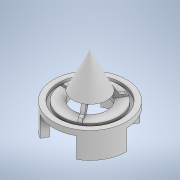
# Autodesk Inventor part: Reflector+feet
Saved by Autodesk Inventor 2022.4 (Build 264492010, 492A)
## iProperties
Created: 2022-12-05
Part Number: Reflector+feet
Material: Generic
Document SubType Name: Modeling
Designer: tmass
Density: 1 g/cm^3
Appearance: Default
Author: tmass
Autodesk Inventor part; units mm, degrees
ref_plane "YZ Plane" through (0, 0, 0) normal (1, 0, 0) x (0, 1, 0)
ref_plane "XY Plane" through (0, 0, 0) normal (0, 0, 1) x (1, 0, 0)
sketch "Sketch1" plane through (0, 0, 0) normal (0, 0, 1) x (1, 0, 0)
  line L0 (0, 60) -> (25, 8)
  line L1 (25, 8) -> (0, -5)
  line L2 (0, -5) -> (0, 0)
  line L3 (0, 0) -> (0, 60)
  dimension "d1" = 60
  dimension "d2" = 13
  dimension "d18" = 5
  dimension "d19" = 25
  constraints: 8 end point, 1 collinear, 1 vertical
  measures "d1" distance of L0.start L2.end
  measures "d2" vertical distance of L1.end L0.end
  measures "d18" distance of L1.end L2.end
  measures "d19" distance from line of L3 L0.end
revolve "Revolution1" add sketch "Sketch1" angle 360 about axis through (0, 0, 0) along (0, 1, 0)
ref_plane "Work Plane1" through (0, -5, 0) normal (0, 1, 0) x (-1, 0, 0)
sketch "Sketch3" plane through (0, -5, 0) normal (0, 1, 0) x (-1, 0, 0)
  circle A0 centre (0, 0) radius 25
  circle A1 centre (0, 0) radius 41.25
  dimension "d7" = 50
  dimension "d8" = 82.5
  constraints: 2 centre point, 2 coincident
  measures "d7" diameter of A0
  measures "d8" diameter of A1
extrude "Extrusion1" add sketch "Sketch3" against normal blind 8
sketch "Sketch4" plane through (0, 0, 0) normal (0, 0, 1) x (1, 0, 0)
  line L0 (0, 60) -> (-25, 8) projected
  line L1 (41.25, -5) -> (-41.25, -5) projected
  line L2 (-25, -13) -> (-25, -5) projected
  line L3 (25, -13) -> (25, -5) projected
  line L4 (41.25, -5) -> (41.25, -13) projected
  line L5 (-41.25, -5) -> (-41.25, -13) projected
  line L6 (25, 8) -> (0, -5) projected
  line L7 (0, 60) -> (25, 8) projected
  line L8 (-37.2957, -1.4547) -> (-41.25, -5)
  line L9 (-25, -5) -> (-15.8228, 3.2278)
  line L10 (-41.25, -5) -> (-25, -5)
  line L11 (-25, 8) -> (25, 8) projected
  line L12 (-25, 8) -> (-12.5712, 19.143)
  line L13 (-12.5712, 19.143) -> (-7.4345, 10.7484)
  line L14 (-7.4345, 10.7484) -> (-15.8228, 3.2278)
  line L15 (-25, 8) -> (-30.5847, -1.4547)
  line L16 (-37.2957, -1.4547) -> (-30.5847, -1.4547)
  point P0 (0, 0)
  point P1 (0, -5)
  point P2 (-10.5, 8)
  constraints: 16 end point, 2 collinear, 2 parallel, 1 horizontal, 1 other
extrude "Extrusion2" add sketch "Sketch4" along normal mid plane 5 contours L11 L14 L9 L1 L8 L16 L15
pattern_circular "Circular Pattern1" count 3 over 360 about axis through (0, -10, 0) along (0, 1, 0) of "Extrusion2"
sketch "Sketch5" plane through (0, -5, 0) normal (0, 1, 0) x (1, 0, 0)
  circle A0 centre (0, 0) radius 39.5
  circle A1 centre (0, 0) radius 28.5
  dimension "d16" = 79
  dimension "d17" = 57
  constraints: 2 centre point, 2 coincident
  measures "d16" diameter of A0
  measures "d17" diameter of A1
sketch "Sketch6" plane through (0, -5, 0) normal (0, 1, 0) x (1, 0, 0)
  circle A0 centre (0, 0) radius 41.25
  circle A1 centre (0, 0) radius 45.75
  circle A2 centre (0, 0) radius 53.5003
  dimension "d20" = 82.5
  dimension "d21" = 4.5
  constraints: 3 centre point, 3 coincident
  measures "d20" diameter of A0
  measures "d21" radial gap between concentric circles of A0 A1
extrude "Extrusion3" add sketch "Sketch6" against normal blind 8 contours A1 | A2
sketch "Sketch7" plane through (0, -5, 0) normal (0, 1, 0) x (1, 0, 0)
  circle A0 centre (0, 0) radius 45.75 projected
  circle A1 centre (0, 0) radius 41.25 projected
extrude "Extrusion4" cut sketch "Sketch7" against normal blind 4
sketch "Sketch8" plane through (0, -13, 0) normal (0, -1, 0) x (1, 0, 0)
  circle A0 centre (0, 0) radius 53.5003
  circle A1 centre (0, 0) radius 53.5003 projected
  circle A2 centre (0, 0) radius 43.5003
  line L0 (0, -60.7067) -> (0, 74.3031)
  line L1 (53.5003, -65.9653) -> (53.5003, 59.8233)
  line L2 (-62.5744, 0) -> (102.4614, 0)
  line L3 (-37.8313, -65.5258) -> (42.3793, 73.4032)
  line L4 (39.8021, -68.9393) -> (-31.97, 55.3736)
  point P0 (26.7502, 46.3326)
  point P1 (21.7502, 37.6724)
  point P2 (43.5003, 0)
  point P3 (53.5003, 0)
  point P4 (-21.7502, -37.6724)
  point P5 (-26.7502, -46.3326)
  point P6 (26.7502, -46.3326)
  point P7 (21.7502, -37.6724)
  point P8 (-21.7502, 37.6724)
  point P9 (-26.7502, 46.3326)
  point P10 (-53.5003, 0)
  point P11 (-43.5003, 0)
  dimension "d26" = 0
  dimension "d27" = 10
  dimension "d28" = 120
  dimension "d29" = 120
  dimension "d30" = 120
  constraints: 10 end point, 2 centre point, 2 coincident, 2 point on line, 1 horizontal, 1 perpendicular, 1 tangent, 1 vertical
  measures "d26" radial gap between concentric circles of A0 A1
  measures "d27" radial gap between concentric circles of A0 A2
  measures "d28" angle of L2 L4
  measures "d29" angle of L2 L3
  measures "d30" angle of L4 L3
extrude "Extrusion5" add sketch "Sketch8" along normal blind 30 contours L2 A2 L3 A0 | A0 L0 A2 L4 | A0 L3 A2 L0 | L4 A2 L2 A0 picked at (40.4215, 23.3374) picked at (5.6147, -49.6757) picked at (-3.0967, -49.896) picked at (-40.4215, 23.3374)
equation "\"d29\" = d28"
body "Solid1"
